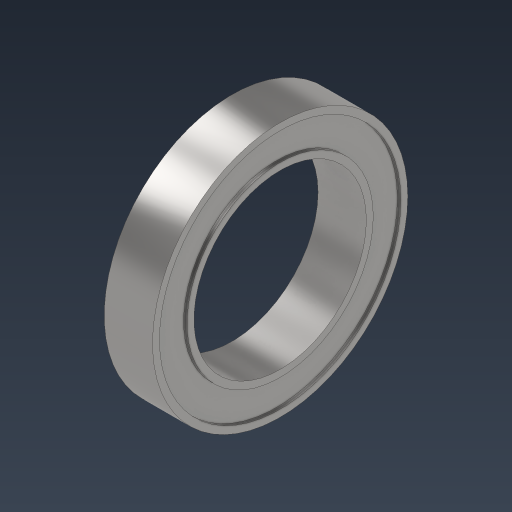
# Autodesk Inventor part: 6805
Saved by Autodesk Inventor 2024.1 (Build 281209000, 209)
## iProperties
Created: 2024-01-12
Part Number: 6805
Material: Stainless Steel
Document SubType Name: Modeling
Designer: dzw04
Density: 8 g/cm^3
Appearance: Semi-Polished
Author: dzw04
Autodesk Inventor part; units mm, degrees
ref_plane "YZ Plane" through (0, 0, 0) normal (1, 0, 0) x (0, 1, 0)
ref_plane "XZ Plane" through (0, 0, 0) normal (0, 1, 0) x (-1, 0, 0)
ref_plane "XY Plane" through (0, 0, 0) normal (0, 0, 1) x (1, 0, 0)
sketch "Sketch1" plane through (0, 0, 0) normal (0, 1, 0) x (-1, 0, 0)
  line L0 (0, 0) -> (0, -12.5) construction
  line L1 (0, -12.5) -> (7, -12.5)
  line L2 (7, -12.5) -> (7, -13.5)
  line L3 (7, -13.5) -> (0, -13.5)
  line L4 (0, -13.5) -> (0, -12.5)
  line L5 (3.5, -13.5) -> (3.5, -17.5) construction
  line L6 (0, -17.5) -> (7, -17.5)
  line L7 (7, -17.5) -> (7, -18.5)
  line L8 (7, -18.5) -> (0, -18.5)
  line L9 (0, -18.5) -> (0, -17.5)
  line L10 (0, 0) -> (7, 0)
  line L11 (0.5, -13.5) -> (6.5, -13.5)
  line L12 (6.5, -13.5) -> (6.5, -17.5)
  line L13 (6.5, -17.5) -> (0.5, -17.5)
  line L14 (0.5, -17.5) -> (0.5, -13.5)
  line L15 (0.5, -13.5) -> (6.5, -17.5) construction
  line L16 (6.5, -13.5) -> (0.5, -17.5) construction
  point P0 (3.5, -15.5)
  point P1 (0.5, -17.5)
  dimension "d0" = 12.5
  dimension "d1" = 7
  dimension "d2" = 1
  dimension "d3" = 4
  dimension "d4" = 7
  dimension "d5" = 1
  dimension "d6" = 7
  dimension "d7" = 6
  dimension "d8" = 4
  constraints: 34 end point, 6 parallel, 5 midpoint, 4 horizontal, 3 perpendicular, 2 vertical
  measures "d0" distance of L0.start L0.end
  measures "d1" distance of L2.end L3.end
  measures "d2" distance of L1.end L2.end
  measures "d3" distance of L5.end L5.start
  measures "d4" distance of L7.end L8.end
  measures "d5" distance of L6.end L7.end
  measures "d6" distance of L0.start L10.end
  measures "d7" distance of L12.end L13.end
  measures "d8" distance of L11.end L12.end
revolve "Revolution1" add sketch "Sketch1" angle 360 about axis through (0, 0, 0) along (-1, 0, 0)
equation "\"d8\" = d3"
body "Solid1"
